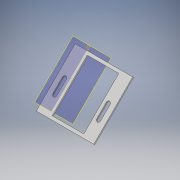
# Autodesk Inventor part: 20_Cube_Insert_Beamsplittercube_Dichroicmirror_Retainplate
Saved by Autodesk Inventor 2019 (Build 230136000, 136)
## iProperties
Created: 2019-08-12
Part Number: 20_Cube_Insert_Beamsplittercube_Dichroicmirror_Retainplate
Material: Generic
Document SubType Name: Modeling
Designer: diederichbenedict
Density: 1 g/cm^3
Appearance: Default
Author: diederichbenedict
Autodesk Inventor part; units mm, degrees
ref_plane "YZ Plane" through (0, 0, 0) normal (1, 0, 0) x (0, 1, 0)
ref_plane "XZ Plane" through (0, 0, 0) normal (0, 1, 0) x (-1, 0, 0)
ref_plane "XY Plane" through (0, 0, 0) normal (0, 0, 1) x (1, 0, 0)
ref_plane "Work Plane2" through (-65.3804, 18.9113, -35.9508) normal (-1, 0, 0) x (0, -0.7071, -0.7071)
ref_plane "Work Plane3" through (-52.8804, 7.2095, -21.4206) normal (0, 0.7071, 0.7071) x (-1, 0, 0)
sketch "Sketch3" plane through (-52.8804, 7.2095, -21.4206) normal (0, 0.7071, 0.7071) x (-1, 0, 0)
  circle A0 centre (16, 5.6569) radius 1.4 construction
  circle A1 centre (-16, 5.6569) radius 1.4 construction
  line L0 (-16.9, -3.0998) -> (-16.9, -27) construction
  line L1 (14.3, 19.8) -> (12.8, 19.8) construction
  line L2 (14.3, 19.8) -> (14.3, -19.254) construction
  line L3 (12.8, 19.8) -> (12.8, -18.254) construction
  line L4 (-12.8, -18.254) -> (-12.8, 19.8) construction
  line L5 (-12.8, 19.8) -> (-14.3, 19.8) construction
  line L6 (-14.3, 19.8) -> (-14.3, -18.254) construction
  line L7 (12.8, -18.254) -> (-12.8, -18.254) construction
  line L8 (-12.5, -18.5487) -> (12.5, -18.5487) construction
  line L9 (18, -17.4431) -> (-18, -17.4431)
  line L10 (-18, -17.4431) -> (-18, 22.7569)
  line L11 (-18, 22.7569) -> (18, 22.7569)
  line L12 (18, 22.7569) -> (18, -17.4431)
  line L13 (10.8, -15.4431) -> (-12.3, -15.4431)
  line L14 (-12.3, -15.4431) -> (-12.3, 20.7569)
  line L15 (-12.3, 20.7569) -> (10.8, 20.7569)
  line L16 (10.8, 20.7569) -> (10.8, -15.4431)
  circle A2 centre (16, 5.6569) radius 1.4
  circle A3 centre (-16, 5.6569) radius 1.4
  line L17 (16, 10.5407) -> (16, 0.773) construction
  line L18 (14.6, 10.5407) -> (14.6, 0.773)
  line L19 (17.4, 0.773) -> (17.4, 10.5407)
  arc A4 (17.4, 10.5407) -> (14.6, 10.5407) centre (16, 10.5407) ccw
  arc A5 (14.6, 0.773) -> (17.4, 0.773) centre (16, 0.773) ccw
  line L20 (-16, 10.5407) -> (-16, 0.773) construction
  line L21 (-17.4, 10.5407) -> (-17.4, 0.773)
  line L22 (-14.6, 0.773) -> (-14.6, 10.5407)
  arc A6 (-14.6, 10.5407) -> (-17.4, 10.5407) centre (-16, 10.5407) ccw
  arc A7 (-17.4, 0.773) -> (-14.6, 0.773) centre (-16, 0.773) ccw
  point P0 (-52.8804, 20.2446)
  dimension "d12" = 2
  dimension "d13" = 2
  dimension "d14" = 23.1
  dimension "d15" = 17.1
  dimension "d16" = 2
  dimension "d17" = 2
  dimension "d18" = 2
  dimension "d19" = 2
  constraints: 50 end point, 8 centre point, 8 point on circle, 8 tangent, 7 parallel, 6 horizontal, 6 vertical, 2 coincident, 2 concentric, 2 midpoint, 2 perpendicular, 16 other
  measures "d12" distance from line of L12 A0.centre
  measures "d13" distance from line of A1.centre L10
  measures "d14" distance from line of L9 A1.centre
  measures "d15" distance from line of L11 A1.centre
  measures "d16" distance between parallel lines of L3 L16
  measures "d17" distance between parallel lines of L6 L14
  measures "d18" distance between parallel lines of L13 L9
  measures "d19" distance between parallel lines of L11 L15
extrude "Extrusion3" add sketch "Sketch3" along normal blind 1
sketch "Sketch4" plane through (-52.8804, 7.2095, -21.4206) normal (0, -0.7071, -0.7071) x (-1, 0, 0)
  line L0 (-12.3, 15.4431) -> (-12.3, -20.7569) projected
  line L1 (-12.3, -20.7569) -> (10.8, -20.7569) projected
  line L2 (10.8, -20.7569) -> (10.8, 15.4431) projected
  line L3 (10.8, 15.4431) -> (-12.3, 15.4431) projected
  line L4 (-18, 17.4431) -> (18, 17.4431) projected
  line L5 (18, 17.4431) -> (18, -22.7569) projected
  line L6 (18, -22.7569) -> (-18, -22.7569) projected
  line L7 (-18, -22.7569) -> (-18, 17.4431) projected
  line L8 (-18, 17.4431) -> (18, 17.4431) projected
  line L9 (-12.3, 15.4431) -> (10.8, 15.4431) projected
  line L10 (9.607, 17.4431) -> (-11.0714, 17.4431)
  line L11 (-11.0714, 17.4431) -> (-11.0714, 15.4431)
  line L12 (-11.0714, 15.4431) -> (9.607, 15.4431)
  line L13 (9.607, 15.4431) -> (9.607, 17.4431)
  line L14 (10.8, -20.7569) -> (-12.3, -20.7569) projected
  line L15 (9.607, -22.7569) -> (-11.0714, -22.7569)
  line L16 (-11.0714, -22.7569) -> (-11.0714, -20.7569)
  line L17 (-11.0714, -20.7569) -> (9.607, -20.7569)
  line L18 (9.607, -20.7569) -> (9.607, -22.7569)
  point P0 (-52.8804, -20.2446)
  constraints: 16 end point, 6 point on line, 4 parallel, 2 horizontal, 2 perpendicular
extrude "Extrusion4" add sketch "Sketch4" along normal blind 1 contours L11 L4 L13 L3 | L1 L18 L6 L16
sketch "Sketch5" plane through (-52.8804, 7.2095, -21.4206) normal (0, -0.7071, -0.7071) x (-1, 0, 0)
  line L0 (-18, 17.4431) -> (18, 17.4431) projected
  line L1 (18, -22.7569) -> (-18, -22.7569) projected
  line L2 (-18, -22.7569) -> (-21, -22.7569)
  line L3 (-21, -22.7569) -> (-21, 17.4431)
  line L4 (-21, 17.4431) -> (-18, 17.4431)
  line L5 (-18, 17.4431) -> (-18, -22.7569)
  line L6 (18, -22.7569) -> (21, -22.7569)
  line L7 (21, -22.7569) -> (21, 17.4431)
  line L8 (21, 17.4431) -> (18, 17.4431)
  line L9 (18, 17.4431) -> (18, -22.7569)
  point P0 (-52.8804, -20.2446)
  dimension "d24" = 3
  dimension "d25" = 3
  dimension "d28" = 40.2
  constraints: 16 end point, 4 parallel, 2 horizontal, 2 perpendicular, 2 point on line
  measures "d24" distance of L3.end L4.end
  measures "d25" distance of L8.end L7.end
  measures "d28" distance of L2.end L3.end
extrude "Extrusion5" add sketch "Sketch5" against normal up to surface (1 mm away) contours L5 L2 L3 L4 | L8 L7 L6 L9
body "Solid2"
